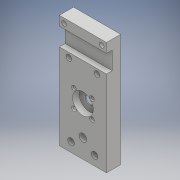
# Autodesk Inventor part: Base_moteur
Saved by Autodesk Inventor 2018 (Build 220112000, 112)
## iProperties
Created: 2019-10-30
Part Number: Base_moteur
Material: Generic
Document SubType Name: Modeling
Designer: hugo
Density: 1 g/cm^3
Appearance: Default
Author: hugo
Autodesk Inventor part; units mm, degrees
ref_plane "YZ Plane" through (0, 0, 0) normal (1, 0, 0) x (0, 1, 0)
ref_plane "XZ Plane" through (0, 0, 0) normal (0, 1, 0) x (-1, 0, 0)
ref_plane "XY Plane" through (0, 0, 0) normal (0, 0, 1) x (1, 0, 0)
sketch "Sketch1" plane through (0, 0, 0) normal (0, 1, 0) x (-1, 0, 0)
  line L0 (0, 0) -> (50, 0)
  line L1 (50, 0) -> (50, -120)
  line L2 (50, -120) -> (0, -120)
  line L3 (0, -120) -> (0, 0)
  dimension "d0" = 50
  dimension "d1" = 120
  constraints: 8 end point, 2 parallel, 1 horizontal, 1 perpendicular
  measures "d0" distance of L1.end L2.end
  measures "d1" distance of L0.end L1.end
extrude "Extrusion1" add sketch "Sketch1" along normal blind 15
sketch "Sketch2" plane through (0, 15, 0) normal (0, 1, 0) x (1, 0, 0)
  circle A0 centre (-5, 5) radius 2.5
  line L0 (0, 0) -> (0, 120) projected
  line L1 (-50, 0) -> (0, 0) projected
  line L2 (-25, 0) -> (-25, 120) construction
  line L3 (0, 120) -> (-50, 120) construction
  circle A1 centre (-12.5, 110) radius 3.5
  circle A2 centre (-45, 5) radius 2.5
  circle A3 centre (-37.5, 110) radius 3.5
  dimension "d4" = 5
  dimension "d5" = 5
  dimension "d6" = 5
  dimension "d7" = 7
  dimension "d8" = 10
  dimension "d9" = 12.5
  constraints: 4 centre point, 2 end point, 2 midpoint, 2 symmetric about line, 2 other
  measures "d4" diameter of A0
  measures "d5" distance from line of L0 A0.centre
  measures "d6" distance from line of L1 A0.centre
  measures "d7" diameter of A1
  measures "d8" distance from line of L3 A1.centre
  measures "d9" distance from line of L0 A1.centre
extrude "Extrusion2" cut sketch "Sketch2" against normal blind 20
sketch "Sketch3" plane through (0, 15, 0) normal (0, 1, 0) x (1, 0, 0)
  circle A0 centre (-37.5, 110) radius 3.5 projected
  circle A1 centre (-12.5, 110) radius 3.5 projected
  circle A2 centre (-25, 62.5) radius 22.5
  point P0 (0, 0)
  dimension "d12" = 45
  dimension "d13" = 47.5
  constraints: 1 centre point
  measures "d12" diameter of A2
  measures "d13" vertical distance of A1.centre A2.centre
extrude "Extrusion3" cut sketch "Sketch3" against normal blind 5.5 contours A2
sketch "Sketch4" plane through (-25, 9.5, -62.5) normal (0, 1, 0) x (1, 0, 0)
  circle A0 centre (0, 0) radius 22.5 projected
  circle A1 centre (0, 6.3) radius 9.5
  point P0 (25, -62.5)
  dimension "d16" = 19
  dimension "d17" = 6.3
  constraints: 1 centre point
  measures "d16" diameter of A1
  measures "d17" distance of A1.centre A0.centre
extrude "Extrusion4" cut sketch "Sketch4" against normal blind 1.7 contours A1
sketch "Sketch5" plane through (-25, 7.8, -68.8) normal (0, 1, 0) x (1, 0, 0)
  circle A0 centre (0, 0) radius 4.5
  point P0 (25, -68.8)
  dimension "d20" = 9
  constraints: 1 centre point
  measures "d20" diameter of A0
extrude "Extrusion5" cut sketch "Sketch5" against normal up to next
sketch "Sketch7" plane through (0, 0, 0) normal (0, -1, 0) x (1, 0, 0)
  circle A0 centre (-25, -68.8) radius 4.5 projected
  circle A1 centre (-25, -68.8) radius 11
  point P0 (0, 0)
  dimension "d35" = 22
  constraints: 1 centre point, 1 coincident
  measures "d35" diameter of A1
extrude "Extrusion7" cut sketch "Sketch7" against normal blind 7
sketch "Sketch8" plane through (0, 0, 0) normal (0, -1, 0) x (1, 0, 0)
  circle A0 centre (-25, -68.8) radius 4.5 projected
  line L0 (-25, -68.8) -> (-41.3044, -68.8) construction
  line L1 (-25, -68.8) -> (-38.0378, -81.8378) construction
  circle A1 centre (-25, -68.8) radius 13.5 construction
  point P0 (0, 0)
  point P1 (-34.5459, -78.3459)
  point P2 (-15.4541, -78.3459)
  point P3 (-15.4541, -59.2541)
  point P4 (-34.5459, -59.2541)
  dimension "d39" = 27
  dimension "d38" = 45
  dimension "d42" = 360
  constraints: 4 end point, 1 coincident, 1 horizontal, 1 point on line, 8 other
  measures "d38" angle of L1 L0
hole "Hole1" at (-34.5459, 0, -78.3459) at (-15.4541, 0, -78.3459) at (-15.4541, 0, -59.2541) at (-34.5459, 0, -59.2541) direction (0, 1, 0) diameter 3 end through all countersink diameter 5 countersink angle 90
sketch "Sketch10" plane through (0, 15, 0) normal (0, 1, 0) x (1, 0, 0)
  line L0 (-50, 0) -> (-50, 120) projected
  line L1 (-50, 39) -> (0, 39) construction
  circle A0 centre (-25, 68.8) radius 4.5 projected
  line L2 (-50, 29) -> (0, 29) construction
  line L3 (0, 120) -> (0, 0) projected
  line L4 (0, 0) -> (-50, 0) construction
  line L5 (-25, 0) -> (-25, 120) construction
  line L6 (-50, 120) -> (0, 120) construction
  point P0 (-10, 34)
  point P1 (-40, 34)
  dimension "d53" = 29.8
  dimension "d54" = 10
  dimension "d55" = 5
  dimension "d56" = 10
  constraints: 6 end point, 3 point on line, 2 horizontal, 2 midpoint, 1 symmetric about line
  measures "d53" distance from line of A0.centre L1
  measures "d54" distance between parallel lines of L1 L2
  measures "d55" distance from line of L1 point (-10, 34)
  measures "d56" distance from line of L3 point (-10, 34)
hole "Hole2" at (-10, 15, -34) at (-40, 15, -34) direction (0, -1, 0) diameter 6 end through all counterbore diameter 15 counterbore depth 8
sketch "Sketch11" plane through (0, 0, 0) normal (1, 0, 0) x (0, 0, -1)
  line L0 (26.5, 15) -> (41.5, 15) projected
  line L1 (41.5, 7) -> (26.5, 7) projected
  line L2 (7.5, 0) -> (2.5, 0) projected
  line L3 (2.5, 15) -> (7.5, 15) projected
  line L4 (7.5, 0) -> (2.5, 0) projected
  line L5 (2.5, 15) -> (7.5, 15) projected
  line L6 (120, 0) -> (0, 0) projected
  line L7 (2.5, 15) -> (7.5, 15) projected
  line L8 (26.5, 15) -> (41.5, 15) projected
  line L9 (0, 15) -> (120, 15) projected
  line L10 (37, 7) -> (31, 7) projected
  line L11 (41.5, 7) -> (26.5, 7) projected
  line L12 (10, 0) -> (29, 0)
  line L13 (29, 0) -> (29, 6)
  line L14 (29, 6) -> (10, 6)
  line L15 (10, 6) -> (10, 0)
  point P0 (29, 7)
  point P1 (5, 15)
  point P2 (34, 15)
  dimension "d88" = 5
  dimension "d89" = 5
  dimension "d90" = 1
  constraints: 8 end point, 2 parallel, 1 horizontal, 1 midpoint, 1 perpendicular, 1 point on line, 3 other
  measures "d88" distance from line of point (34, 15) L13
  measures "d89" distance from line of L15 point (5, 15)
  measures "d90" distance between parallel lines of L1 L14
extrude "Extrusion8" cut sketch "Sketch11" against normal up to next
sketch "Sketch14" plane through (0, 15, 0) normal (0, 1, 0) x (1, 0, 0)
  circle A0 centre (-37.5, 110) radius 3.5 projected
  circle A1 centre (-25, 100) radius 4
  point P0 (0, 0)
  dimension "d79" = 8
  dimension "d80" = 10
  constraints: 1 centre point
  measures "d79" diameter of A1
  measures "d80" vertical distance of A0.centre A1.centre
extrude "Extrusion11" cut sketch "Sketch14" against normal up to next contours A1
sketch "Sketch15" plane through (0, 15, 0) normal (0, 1, 0) x (1, 0, 0)
  circle A0 centre (-40, 34) radius 3 projected
  circle A1 centre (-25, 100) radius 4 projected
  circle A2 centre (-10, 34) radius 7.5 projected
  circle A3 centre (-40, 34) radius 7.5 projected
  circle A4 centre (-25, 62.5) radius 22.5 projected
  circle A5 centre (-12.5, 110) radius 3.5 projected
  circle A6 centre (-5, 5) radius 2.5 projected
  circle A7 centre (-45, 5) radius 2.5 projected
  circle A8 centre (-37.5, 110) radius 3.5 projected
  line L0 (-50, 0) -> (0, 0) projected
  line L1 (0, 0) -> (0, 120) projected
  line L2 (0, 120) -> (-50, 120) projected
  line L3 (-50, 120) -> (-50, 0) projected
  circle A9 centre (-25, 34) radius 2.5
  dimension "d83" = 5
  constraints: 1 centre point
  measures "d83" diameter of A9
extrude "Extrusion12" cut sketch "Sketch15" against normal blind 8 contours A9
equation "\"d0\" = Hh"
equation "\"d1\" = Lh"
equation "\"d2\" = lh"
equation "\"d9\" = 0.25 * Hh"
equation "\"d54\" = lB"
equation "\"d55\" = 0.5 * d54"
equation "\"Hh\" = 50"
equation "\"Lh\" = 120"
equation "\"lh\" = 15"
equation "\"lB\" = 10"
equation "\"lr\" = 1.8"
body "Solid1"
